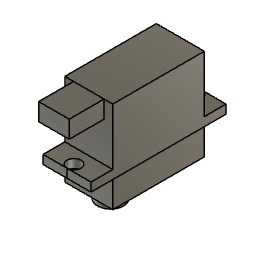
DS386 v4 (Autodesk Fusion 360 design; units mm, degrees)
Autodesk Fusion 360 part; units mm, degrees
sketch "Sketch1" plane through (0, 0, 0) normal (0, 0, 1) x (1, 0, 0)
  line L0 (0, 0) -> (11, 0)
  line L1 (11, 0) -> (11, -21)
  line L2 (11, -21) -> (0, -21)
  line L3 (0, -21) -> (0, 0)
  constraint horizontal L0
  constraint vertical L1
  constraint horizontal L2
  constraint vertical L3
  constraint coincident L0.start L3.end
extrude "Extrude1" add sketch "Sketch1" along normal blind 13 makes body 1
sketch "Sketch2" plane through (0, 0, 0) normal (0, 0, -1) x (1, 0, 0)
  line L0 (11, 21) -> (0, 21)
  line L1 (0, 21) -> (0, 0)
  line L2 (0, 0) -> (11, 0)
  line L3 (11, 0) -> (11, 21)
  line L4 (0, -5) -> (11, -5)
  line L5 (11, -5) -> (11, 26)
  line L6 (11, 26) -> (0, 26)
  line L7 (0, 26) -> (0, -5)
  dimension "d3" = 11
  constraint horizontal L4
  constraint vertical L5
  constraint horizontal L6
  constraint vertical L7
  measures "d3" distance of L4.start L4.end
extrude "Extrude2" add sketch "Sketch2" along normal blind 2 bodies 1
sketch "Sketch3" plane through (0, 0, -2) normal (0, 0, -1) x (1, 0, 0)
  line L0 (0, 26) -> (0, -5)
  line L1 (0, -5) -> (11, -5)
  line L2 (11, -5) -> (11, 26)
  line L3 (11, 26) -> (0, 26)
  circle A0 centre (5.5, -3.4) radius 1.6
  circle A1 centre (5.5, 24.4) radius 1.6
  dimension "d6" = 3.2
  dimension "d7" = 5.5
  dimension "d8" = 5.5
  dimension "d9" = 1.6
  dimension "d10" = 1.6
  dimension "d11" = 3.2
  measures "d6" diameter of A1
  measures "d7" distance of L2 A1.centre
  measures "d8" distance of L2 A0.centre
  measures "d9" distance of L3 A1.centre
  measures "d10" distance of L1 A0.centre
  measures "d11" diameter of A0
extrude "Extrude3" cut sketch "Sketch3" against normal blind 2 contours A0 | A1 bodies 1
sketch "Sketch4" plane through (0, 0, -2) normal (0, 0, -1) x (1, 0, 0)
  line L0 (0, 26) -> (0, -5)
  line L1 (0, -5) -> (5.5, -5)
  circle A0 centre (5.5, -3.4) radius 1.6
  line L2 (5.5, -5) -> (11, -5)
  line L3 (11, -5) -> (11, 26)
  line L4 (11, 26) -> (5.5, 26)
  circle A1 centre (5.5, 24.4) radius 1.6
  line L5 (5.5, 26) -> (0, 26)
  line L6 (0, 0) -> (11, 0)
  line L7 (11, 0) -> (11, 21)
  line L8 (11, 21) -> (0, 21)
  line L9 (0, 21) -> (0, 0)
  constraint horizontal L6
  constraint vertical L7
  constraint horizontal L8
  constraint vertical L9
  constraint coincident L3 L7.end
  constraint coincident L6.start L9.end
extrude "Extrude4" add sketch "Sketch4" along normal blind 6 separate body contours L0 L3 L6 L7 L8 L9 makes body 2
sketch "Sketch5" plane through (0, 0, -8) normal (0, 0, -1) x (1, 0, 0)
  line L0 (0, 21) -> (0, 0)
  line L1 (0, 0) -> (11, 0)
  line L2 (11, 0) -> (11, 21)
  line L3 (11, 21) -> (0, 21)
  circle A0 centre (5.5, 16) radius 3
  dimension "d16" = 6
  dimension "d17" = 5
  measures "d16" diameter of A0
  measures "d17" distance of L3 A0.centre
extrude "Extrude5" add sketch "Sketch5" along normal blind 3 contours A0 bodies 2
sketch "Sketch6" plane through (0, 0, -11) normal (0, 0, -1) x (1, 0, 0)
  circle A0 centre (5.5, 16) radius 3
  circle A1 centre (5.5, 16) radius 1.55
  dimension "d20" = 3.1
  constraint concentric A0 A1
  measures "d20" diameter of A1
extrude "Extrude6" cut sketch "Sketch6" against normal blind 6 contours A1 bodies 2
sketch "Sketch7" plane through (0, 0, 13) normal (0, 0, 1) x (-1, 0, 0)
  line L0 (0, 21) -> (-11, 21)
  line L1 (-11, 21) -> (-11, 0)
  line L2 (-11, 0) -> (0, 0)
  line L3 (0, 0) -> (0, 21)
  line L4 (-9, 21) -> (-2, 21)
  line L5 (-2, 21) -> (-2, 29)
  line L6 (-2, 29) -> (-9, 29)
  line L7 (-9, 29) -> (-9, 21)
  dimension "d23" = 2
  constraint horizontal L4
  constraint vertical L5
  constraint horizontal L6
  constraint vertical L7
  constraint coincident L0 L4.start
  measures "d23" distance of L3 L5
extrude "Extrude7" add sketch "Sketch7" against normal blind 4 separate body contours L0 L4 L5 L6 L7 makes body 3
